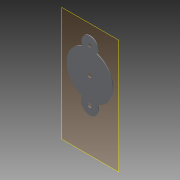
# Autodesk Inventor part: driveGearSupportLayer
Saved by Autodesk Inventor 2013 (Build 170138000, 138)
## iProperties
Created: 2014-07-02
Part Number: driveGearSupportLayer
Material: Generic
Document SubType Name: Modeling
Designer: Nano
Density: 1 g/cm^3
Author: Nano
Autodesk Inventor part; units mm, degrees
ref_plane "YZ Plane" through (0, 0, 0) normal (1, 0, 0) x (0, 1, 0)
ref_plane "XZ Plane" through (0, 0, 0) normal (0, 1, 0) x (-1, 0, 0)
ref_plane "XY Plane" through (0, 0, 0) normal (0, 0, 1) x (1, 0, 0)
ref_plane "Work Plane1" through (0, 0, 0) normal (0, 0, 1) x (1, 0, 0)
sketch "Sketch1" plane through (0, 0, 0) normal (0, 0, 1) x (1, 0, 0)
  arc A0 (-0.6085, 73.7601) -> (-2.2645, 77.2932) centre (0, 76.2) ccw construction
  circle A1 centre (0, 76.2) radius 3.175
  arc A2 (13.8637, 68.3454) -> (-13.8637, 68.3454) centre (0, 76.2) ccw
  circle A3 centre (0, 25.4) radius 3.175 construction
  circle A4 centre (0, -25.4) radius 3.175 construction
  arc A5 (-14.809, -17.2286) -> (14.809, -17.2286) centre (0, -25.4) ccw
  circle A6 centre (0, 25.4) radius 4.1833
  circle A7 centre (0, -25.4) radius 4.0324
  arc A8 (14.809, -17.2286) -> (13.8637, 68.3454) centre (0, 25.4) ccw
  arc A9 (-13.8637, 68.3454) -> (-14.809, -17.2286) centre (0, 25.4) ccw
  point P0 (0, 0)
  dimension "d0" = 6.35
  constraints: 8 point on circle, 7 centre point
  measures "d0" diameter of A1
extrude "Extrusion1" add sketch "Sketch1" along normal blind 1.5875
body "Solid1"
